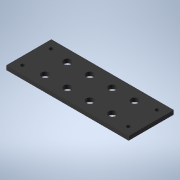
# Autodesk Inventor part: SequenceMachine_VialPlate
Saved by Autodesk Inventor 2022 (Build 260153000, 153)
## iProperties
Created: 2022-07-18
Part Number: SequenceMachine_VialPlate
Material: Generic
Document SubType Name: Modeling
Designer: devon
Density: 1 g/cm^3
Appearance: Default
Author: devon
Autodesk Inventor part; units mm, degrees
ref_plane "YZ Plane" through (0, 0, 0) normal (1, 0, 0) x (0, 1, 0)
ref_plane "XZ Plane" through (0, 0, 0) normal (0, 1, 0) x (-1, 0, 0)
ref_plane "XY Plane" through (0, 0, 0) normal (0, 0, 1) x (1, 0, 0)
sketch "Sketch1" plane through (0, 0, 0) normal (0, 1, 0) x (-1, 0, 0)
  circle A0 centre (0, 0) radius 6.25
  line L0 (0, 0) -> (0, 25.4) construction
  line L1 (0, 0) -> (-101.6, 0) construction
  circle A1 centre (0, 35) radius 6.25
  circle A2 centre (-35, 0) radius 6.25
  circle A3 centre (-35, 35) radius 6.25
  circle A4 centre (-70, 0) radius 6.25
  circle A5 centre (-70, 35) radius 6.25
  circle A6 centre (-105, 0) radius 6.25
  circle A7 centre (-105, 35) radius 6.25
  line L2 (42.9, -17.5) -> (-147.9, -17.5)
  line L3 (-147.9, -17.5) -> (-147.9, 52.5)
  line L4 (-147.9, 52.5) -> (42.9, 52.5)
  line L5 (42.9, 52.5) -> (42.9, -17.5)
  circle A8 centre (30.2, -4.8) radius 3.302
  circle A9 centre (-135.2, -4.8) radius 3.302
  circle A10 centre (-135.2, 39.8) radius 3.302
  circle A11 centre (30.2, 39.8) radius 3.302
  dimension "d0" = 12.5
  dimension "d1" = 25.4
  dimension "d2" = 101.6
  dimension "d5" = 35
  dimension "d8" = 35
  dimension "d11" = 42.9
  dimension "d12" = 42.9
  dimension "d13" = 17.5
  dimension "d14" = 17.5
  dimension "d15" = 6.604
  dimension "d16" = 12.7
  dimension "d17" = 12.7
  dimension "d18" = 6.604
  dimension "d19" = 12.7
  dimension "d20" = 6.604
  dimension "d21" = 12.7
  dimension "d22" = 6.604
  constraints: 12 centre point, 12 end point, 3 horizontal, 2 parallel, 2 vertical, 1 coincident, 1 perpendicular, 14 other
  measures "d0" diameter of A0
  measures "d1" distance of L0.start L0.end
  measures "d2" distance of L0.start L1.end
  measures "d5" distance of L0.start A1.centre
  measures "d8" distance of L0.start A2.centre
  measures "d11" distance from line of L5 point (0, 0)
  measures "d12" distance from line of A6.centre L3
  measures "d13" distance from line of L2 point (0, 0)
  measures "d14" distance from line of L4 A1.centre
  measures "d15" diameter of A8
  measures "d16" distance from line of L2 A8.centre
  measures "d17" distance from line of L5 A8.centre
  measures "d18" diameter of A9
  measures "d19" distance from line of L3 A9.centre
  measures "d20" diameter of A10
  measures "d21" distance from line of L4 A10.centre
  measures "d22" diameter of A11
extrude "Extrusion1" add sketch "Sketch1" along normal blind 6.35
equation "\"d13\" = 0.5 * d5"
equation "\"d14\" = 0.5 * d5"
body "Solid1"
